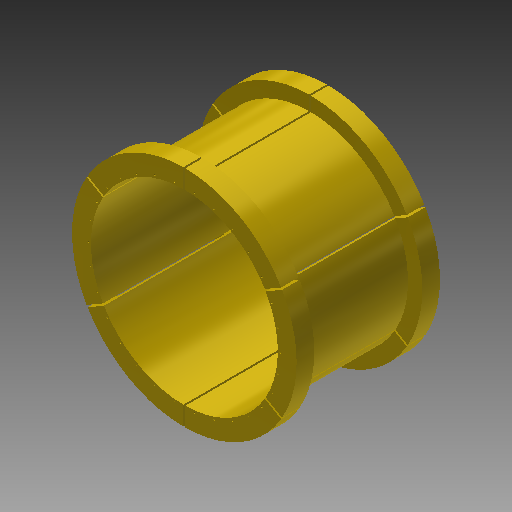
# Autodesk Inventor part: Electrode 4
Saved by Autodesk Inventor 2017 (Build 210142000, 142)
## iProperties
Created: 2009-05-06
Part Number: Electrode 4
Document SubType Name: Modeling
Designer: Serena
Material: Default
Density: 1 g/cm^3
Appearance: Glossy - Gold
Author: Serena
Autodesk Inventor part; units mm, degrees
ref_plane "YZ Plane" through (0, 0, 0) normal (1, 0, 0) x (0, 1, 0)
ref_plane "XZ Plane" through (0, 0, 0) normal (0, 1, 0) x (-1, 0, 0)
ref_plane "XY Plane" through (0, 0, 0) normal (0, 0, 1) x (1, 0, 0)
sketch "Sketch1" plane through (0, 0, 0) normal (0, 0, 1) x (1, 0, 0)
  circle A0 centre (0, 0) radius 100.35
  circle A1 centre (0, 0) radius 105.35
  dimension "d0" = 200.7
  dimension "d1" = 210.7
  constraints: 2 centre point, 1 coincident
  measures "d0" diameter of A0
  measures "d1" diameter of A1
extrude "Extrusion1" add sketch "Sketch1" along normal blind 154
sketch "Sketch2" plane through (0, 0, 154) normal (0, 0, 1) x (1, 0, 0)
  circle A0 centre (0, 0) radius 100.35
  circle A1 centre (0, 0) radius 105.35
  line L0 (0, 0) -> (0, -108.273006)
  line L1 (-1, -100.345017) -> (-1, -105.345254)
  line L2 (1, -100.345017) -> (1, -105.345254)
  line L3 (0, -101.649951) -> (1, -101.649951)
  line L4 (0, -102.197731) -> (-1, -102.197731)
  line L5 (-87.401334, -49.306483) -> (-91.731666, -51.806602)
  line L6 (-86.401334, -51.038534) -> (-90.731666, -53.538652)
  line L7 (-86.401334, 51.038534) -> (-90.731666, 53.538652)
  line L8 (-87.401334, 49.306483) -> (-91.731666, 51.806602)
  line L9 (1, 100.345017) -> (1, 105.345254)
  line L10 (-1, 100.345017) -> (-1, 105.345254)
  line L11 (87.401334, 49.306483) -> (91.731666, 51.806602)
  line L12 (86.401334, 51.038534) -> (90.731666, 53.538652)
  line L13 (86.401334, -51.038534) -> (90.731666, -53.538652)
  line L14 (87.401334, -49.306483) -> (91.731666, -51.806602)
  line L15 (87.401334, 49.306483) -> (91.731666, 51.806602)
  line L16 (86.401334, 51.038534) -> (90.731666, 53.538652)
  line L17 (86.401334, -51.038534) -> (90.731666, -53.538652)
  line L18 (87.401334, -49.306483) -> (91.731666, -51.806602)
  line L19 (-1, -100.345017) -> (-1, -105.345254)
  line L20 (1, -100.345017) -> (1, -105.345254)
  line L21 (-87.401334, -49.306483) -> (-91.731666, -51.806602)
  line L22 (-86.401334, -51.038534) -> (-90.731666, -53.538652)
  line L23 (-86.401334, 51.038534) -> (-90.731666, 53.538652)
  line L24 (-87.401334, 49.306483) -> (-91.731666, 51.806602)
  point P0 (-87.53144, -51.691001)
  point P1 (-89.005831, -50.23284)
  point P2 (-88.53144, 49.95895)
  point P3 (-88.005831, 51.964891)
  point P4 (-1, 101.649951)
  point P5 (1, 102.197731)
  point P6 (87.53144, 51.691001)
  point P7 (89.005831, 50.23284)
  point P8 (88.53144, -49.95895)
  point P9 (88.005831, -51.964891)
  point P10 (89.005831, 50.23284)
  point P11 (87.53144, 51.691001)
  point P12 (88.005831, -51.964891)
  point P13 (88.53144, -49.95895)
  point P14 (-1, -102.197731)
  point P15 (1, -101.649951)
  point P16 (-89.005831, -50.23284)
  point P17 (-87.53144, -51.691001)
  point P18 (-88.005831, 51.964891)
  point P19 (-88.53144, 49.95895)
  dimension "d5" = 1
  dimension "d8" = 360
  dimension "d12" = 360
  constraints: 50 end point, 24 point on line, 4 point on circle, 3 parallel, 2 perpendicular, 1 vertical, 104 other
  measures "d5" distance between parallel lines of L1 L0
sketch "Sketch3" plane through (0, 0, 154) normal (0, 0, 1) x (1, 0, 0)
  circle A0 centre (0, 0) radius 100.35
  circle A1 centre (0, 0) radius 105.35
  line L0 (86.401334, -51.038534) -> (90.731666, -53.538652)
  line L1 (87.401334, -49.306483) -> (91.731666, -51.806602)
  line L2 (86.401334, -51.038534) -> (90.731666, -53.538652)
  line L3 (87.401334, -49.306483) -> (91.731666, -51.806602)
  arc A2 (90.731666, -53.538652) -> (91.731666, -51.806602) centre (1.73213, -1.000046) ccw
  arc A3 (86.401334, -51.038534) -> (87.401334, -49.306483) centre (0, 0) ccw
  constraints: 4 end point, 4 point on circle, 2 centre point, 2 collinear
extrude "Extrusion2" cut sketch "Sketch3" against normal blind 155 contours A0 L1 A1 L0 picked at (88.734946, -50.333043)
pattern_circular "Circular Pattern1" count 6 over 360 about axis through (0, 0, 0) along (0, 0, 1) of "Extrusion2"
sketch "Sketch7" plane through (0, 0, 0) normal (0, 0, -1) x (-1, 0, 0)
  arc A0 (1, -100.345017) -> (86.401334, -51.038534) centre (0, 0) ccw
  circle A1 centre (0, 0) radius 103.35
  circle A2 centre (0, 0) radius 120.65
  dimension "d37" = 206.7
  dimension "d38" = 241.3
  constraints: 2 centre point, 2 coincident
  measures "d37" diameter of A1
  measures "d38" diameter of A2
extrude "Extrusion4" add sketch "Sketch7" against normal blind 18.9992
sketch "Sketch6" plane through (0, 0, 154) normal (0, 0, 1) x (1, 0, 0)
  arc A0 (-91.731666, 51.806602) -> (-91.731666, -51.806602) centre (0, 0) ccw
  circle A1 centre (0, 0) radius 120.65
  circle A2 centre (0, 0) radius 103.35
  dimension "d33" = 241.3
  dimension "d34" = 206.7
  constraints: 2 centre point, 2 coincident
  measures "d33" diameter of A1
  measures "d34" diameter of A2
extrude "Extrusion3" add sketch "Sketch6" against normal blind 18.9992
sketch "Sketch4" plane through (0, 0, 0) normal (0, 1, 0) x (-1, 0, 0)
  line L0 (105.35, 0) -> (105.35, 154)
  line L1 (100.35, 0) -> (100.35, 154)
  line L2 (87.401334, 154) -> (100.35, 154)
  line L3 (91.731666, 154) -> (105.35, 154)
  line L4 (102.85, 154) -> (102.85, 142)
  line L5 (102.85, 154) -> (102.85, 162)
  circle A0 centre (102.85, 154.5) radius 1
  line L6 (102.85, 154) -> (102.85, 153.5)
  line L7 (102.85, 154) -> (101.983975, 154)
  line L8 (102.85, 154) -> (103.716025, 154)
  arc A1 (102.85, 153.5) -> (103.716025, 154) centre (102.85, 154.5) ccw
  arc A2 (101.983975, 154) -> (102.85, 153.5) centre (102.85, 154.5) ccw
  line L9 (-1, 0) -> (-1, 154) construction
  line L10 (-86.401334, 154) -> (-1, 154) construction
  line L11 (-86.401334, 154) -> (-86.401334, 0) construction
  line L12 (-1, 0) -> (-86.401334, 0) construction
  line L13 (1, 0) -> (-1, 0) construction
  line L14 (-1, 154) -> (1, 154) construction
  line L15 (1, 135.0008) -> (-1, 135.0008) construction
  line L16 (0, 154) -> (0, 135.0008) construction
  dimension "d20" = 0.5
  dimension "d21" = 2
  dimension "d53" = 102.85
  constraints: 12 end point, 7 point on circle, 5 point on line, 4 concentric, 3 centre point, 2 midpoint, 1 collinear, 1 perpendicular
  measures "d20" distance of L4.start L6.end
  measures "d21" diameter of A0
  measures "d53" distance between parallel lines of L4 L16
revolve "Revolution1" cut sketch "Sketch4" angle 360 about axis through (-102.85, 0, 154) along (0, 0, -1) picked at (103.38639, 153.943623) contours L3 A0 L4
pattern_circular "Circular Pattern2" count 30 over 360 about axis through (0, 0, 0) along (0, 0, 1) of "Revolution1"
sketch "Sketch5" plane through (0, 0, 0) normal (0, 1, 0) x (-1, 0, 0)
  line L0 (105.35, 0) -> (105.35, 154)
  line L1 (100.35, 0) -> (100.35, 154)
  line L2 (91.731666, 0) -> (105.35, 0)
  line L3 (102.85, 0) -> (102.85, 14)
  line L4 (102.85, 0) -> (102.85, -13)
  circle A0 centre (102.85, -0.5) radius 1
  line L5 (102.85, 0) -> (102.85, 0.5)
  line L6 (102.85, 0) -> (101.983975, 0)
  line L7 (102.85, 0) -> (103.716025, 0)
  arc A1 (103.716025, 0) -> (102.85, 0.5) centre (102.85, -0.5) ccw
  arc A2 (102.85, 0.5) -> (101.983975, 0) centre (102.85, -0.5) ccw
  line L8 (1, 0) -> (-1, 0)
  line L9 (-1, 18.9992) -> (1, 18.9992)
  line L10 (0, 0) -> (0, 18.9992) construction
  dimension "d27" = 0.5
  dimension "d28" = 2
  dimension "d54" = 102.85
  constraints: 12 end point, 7 point on circle, 5 point on line, 3 centre point, 3 concentric, 2 midpoint, 1 collinear, 1 perpendicular
  measures "d27" distance of L3.start L5.end
  measures "d28" diameter of A0
  measures "d54" distance between parallel lines of L10 L3
revolve "Revolution2" cut sketch "Sketch5" angle 360 about axis through (-102.85, 0, 0) along (0, 0, 1) picked at (103.38639, 0.056377) contours L3 A0 L2
pattern_circular "Circular Pattern3" count 30 over 360 about axis through (0, 0, 0) along (0, 0, 1) of "Revolution2"
sketch "Sketch8" plane through (0, 0, 0) normal (0, 0, -1) x (-1, 0, 0)
  circle A0 centre (0, 0) radius 120.65
  line L0 (-1, -103.345162) -> (-1, -100.345017)
  arc A1 (-86.401334, -51.038534) -> (-1, -100.345017) centre (0, 0) ccw
  line L1 (-86.401334, -51.038534) -> (-88.999536, -52.538606)
  arc A2 (-89.999536, -50.806556) -> (-88.999536, -52.538606) centre (0, 0) ccw
  line L2 (-89.999536, -50.806556) -> (-87.401334, -49.306483)
  arc A3 (-87.401334, 49.306483) -> (-87.401334, -49.306483) centre (0, 0) ccw
  line L3 (-87.401334, 49.306483) -> (-89.999536, 50.806556)
  arc A4 (-88.999536, 52.538606) -> (-89.999536, 50.806556) centre (0, 0) ccw
  line L4 (-88.999536, 52.538606) -> (-86.401334, 51.038534)
  arc A5 (-1, 100.345017) -> (-86.401334, 51.038534) centre (0, 0) ccw
  line L5 (-1, 100.345017) -> (-1, 103.345162)
  arc A6 (1, 103.345162) -> (-1, 103.345162) centre (0, 0) ccw
  line L6 (1, 103.345162) -> (1, 100.345017)
  arc A7 (86.401334, 51.038534) -> (1, 100.345017) centre (0, 0) ccw
  line L7 (86.401334, 51.038534) -> (88.999536, 52.538606)
  arc A8 (89.999536, 50.806556) -> (88.999536, 52.538606) centre (0, 0) ccw
  line L8 (89.999536, 50.806556) -> (87.401334, 49.306483)
  arc A9 (87.401334, -49.306483) -> (87.401334, 49.306483) centre (0, 0) ccw
  line L9 (87.401334, -49.306483) -> (89.999536, -50.806556)
  arc A10 (88.999536, -52.538606) -> (89.999536, -50.806556) centre (0, 0) ccw
  line L10 (88.999536, -52.538606) -> (86.401334, -51.038534)
  arc A11 (1, -100.345017) -> (86.401334, -51.038534) centre (0, 0) ccw
  line L11 (1, -100.345017) -> (1, -103.345162)
  arc A12 (-1, -103.345162) -> (1, -103.345162) centre (0, 0) ccw
  line L12 (87.401334, -49.306483) -> (104.982376, -59.456902)
  line L13 (86.401334, -51.038534) -> (103.982376, -61.188953)
  constraints: 4 end point, 2 point on circle, 1 parallel, 1 point on line
extrude "Extrusion5" cut sketch "Sketch8" against normal blind 155 contours L13 A10 L12 A0
sketch "Sketch9" plane through (0, 0, 0) normal (0, 0, -1) x (-1, 0, 0)
  line L0 (87.401334, -49.306483) -> (104.982376, -59.456902)
  arc A0 (104.982376, -59.456902) -> (103.982376, -61.188953) centre (0, 0) ccw
  line L1 (103.982376, -61.188953) -> (86.401334, -51.038534)
  arc A1 (1, -100.345017) -> (86.401334, -51.038534) centre (0, 0) ccw
  line L2 (1, -100.345017) -> (1, -103.345162)
  arc A2 (-1, -103.345162) -> (1, -103.345162) centre (0, 0) ccw
  line L3 (-1, -103.345162) -> (-1, -100.345017)
  arc A3 (-86.401334, -51.038534) -> (-1, -100.345017) centre (0, 0) ccw
  line L4 (-86.401334, -51.038534) -> (-88.999536, -52.538606)
  arc A4 (-89.999536, -50.806556) -> (-88.999536, -52.538606) centre (0, 0) ccw
  line L5 (-89.999536, -50.806556) -> (-87.401334, -49.306483)
  arc A5 (-87.401334, 49.306483) -> (-87.401334, -49.306483) centre (0, 0) ccw
  line L6 (-87.401334, 49.306483) -> (-89.999536, 50.806556)
  arc A6 (-88.999536, 52.538606) -> (-89.999536, 50.806556) centre (0, 0) ccw
  line L7 (-88.999536, 52.538606) -> (-86.401334, 51.038534)
  arc A7 (-1, 100.345017) -> (-86.401334, 51.038534) centre (0, 0) ccw
  line L8 (-1, 100.345017) -> (-1, 103.345162)
  arc A8 (1, 103.345162) -> (-1, 103.345162) centre (0, 0) ccw
  line L9 (1, 103.345162) -> (1, 100.345017)
  arc A9 (86.401334, 51.038534) -> (1, 100.345017) centre (0, 0) ccw
  line L10 (86.401334, 51.038534) -> (88.999536, 52.538606)
  arc A10 (89.999536, 50.806556) -> (88.999536, 52.538606) centre (0, 0) ccw
  line L11 (89.999536, 50.806556) -> (87.401334, 49.306483)
  arc A11 (87.401334, -49.306483) -> (87.401334, 49.306483) centre (0, 0) ccw
  line L12 (1, -100.345017) -> (1, -120.645856)
  line L13 (-1, -100.345017) -> (-1, -120.645856)
  constraints: 4 end point, 2 point on circle, 1 parallel, 1 point on line
extrude "Extrusion6" cut sketch "Sketch9" against normal blind 155 contours L13 A2 L12 A0
sketch "Sketch10" plane through (0, 0, 0) normal (0, 0, -1) x (-1, 0, 0)
  line L0 (-1, -120.645856) -> (-1, -100.345017)
  arc A0 (-86.401334, -51.038534) -> (-1, -100.345017) centre (0, 0) ccw
  line L1 (-86.401334, -51.038534) -> (-88.999536, -52.538606)
  arc A1 (-89.999536, -50.806556) -> (-88.999536, -52.538606) centre (0, 0) ccw
  line L2 (-89.999536, -50.806556) -> (-87.401334, -49.306483)
  arc A2 (-87.401334, 49.306483) -> (-87.401334, -49.306483) centre (0, 0) ccw
  line L3 (-87.401334, 49.306483) -> (-89.999536, 50.806556)
  arc A3 (-88.999536, 52.538606) -> (-89.999536, 50.806556) centre (0, 0) ccw
  line L4 (-88.999536, 52.538606) -> (-86.401334, 51.038534)
  arc A4 (-1, 100.345017) -> (-86.401334, 51.038534) centre (0, 0) ccw
  line L5 (-1, 100.345017) -> (-1, 103.345162)
  arc A5 (1, 103.345162) -> (-1, 103.345162) centre (0, 0) ccw
  line L6 (1, 103.345162) -> (1, 100.345017)
  arc A6 (86.401334, 51.038534) -> (1, 100.345017) centre (0, 0) ccw
  line L7 (86.401334, 51.038534) -> (88.999536, 52.538606)
  arc A7 (89.999536, 50.806556) -> (88.999536, 52.538606) centre (0, 0) ccw
  line L8 (89.999536, 50.806556) -> (87.401334, 49.306483)
  arc A8 (87.401334, -49.306483) -> (87.401334, 49.306483) centre (0, 0) ccw
  line L9 (87.401334, -49.306483) -> (104.982376, -59.456902)
  arc A9 (104.982376, -59.456902) -> (-1, -120.645856) centre (0, 0) ccw
  line L10 (86.401334, 51.038534) -> (103.982376, 61.188953)
  line L11 (87.401334, 49.306483) -> (104.982376, 59.456902)
  constraints: 4 end point, 2 parallel, 2 point on circle
extrude "Extrusion7" cut sketch "Sketch10" against normal blind 155 contours A9 L11 A7 L10
sketch "Sketch11" plane through (0, 0, 0) normal (0, 0, -1) x (-1, 0, 0)
  line L0 (86.401334, 51.038534) -> (103.982376, 61.188953)
  arc A0 (103.982376, 61.188953) -> (-1, -120.645856) centre (0, 0) ccw
  line L1 (-1, -120.645856) -> (-1, -100.345017)
  arc A1 (-86.401334, -51.038534) -> (-1, -100.345017) centre (0, 0) ccw
  line L2 (-86.401334, -51.038534) -> (-88.999536, -52.538606)
  arc A2 (-89.999536, -50.806556) -> (-88.999536, -52.538606) centre (0, 0) ccw
  line L3 (-89.999536, -50.806556) -> (-87.401334, -49.306483)
  arc A3 (-87.401334, 49.306483) -> (-87.401334, -49.306483) centre (0, 0) ccw
  line L4 (-87.401334, 49.306483) -> (-89.999536, 50.806556)
  arc A4 (-88.999536, 52.538606) -> (-89.999536, 50.806556) centre (0, 0) ccw
  line L5 (-88.999536, 52.538606) -> (-86.401334, 51.038534)
  arc A5 (-1, 100.345017) -> (-86.401334, 51.038534) centre (0, 0) ccw
  line L6 (-1, 100.345017) -> (-1, 103.345162)
  arc A6 (1, 103.345162) -> (-1, 103.345162) centre (0, 0) ccw
  line L7 (1, 103.345162) -> (1, 100.345017)
  arc A7 (86.401334, 51.038534) -> (1, 100.345017) centre (0, 0) ccw
  line L8 (-1, 100.345017) -> (-1, 120.645856)
  line L9 (1, 100.345017) -> (1, 120.645856)
  constraints: 4 end point, 2 parallel, 2 point on circle
extrude "Extrusion8" cut sketch "Sketch11" against normal blind 155 contours L9 A6 L8 A0
sketch "Sketch12" plane through (0, 0, 0) normal (0, 0, -1) x (-1, 0, 0)
  line L0 (-1, 100.345017) -> (-1, 120.645856)
  arc A0 (-1, 120.645856) -> (-1, -120.645856) centre (0, 0) ccw
  line L1 (-1, -120.645856) -> (-1, -100.345017)
  arc A1 (-86.401334, -51.038534) -> (-1, -100.345017) centre (0, 0) ccw
  line L2 (-86.401334, -51.038534) -> (-88.999536, -52.538606)
  arc A2 (-89.999536, -50.806556) -> (-88.999536, -52.538606) centre (0, 0) ccw
  line L3 (-89.999536, -50.806556) -> (-87.401334, -49.306483)
  arc A3 (-87.401334, 49.306483) -> (-87.401334, -49.306483) centre (0, 0) ccw
  line L4 (-87.401334, 49.306483) -> (-89.999536, 50.806556)
  arc A4 (-88.999536, 52.538606) -> (-89.999536, 50.806556) centre (0, 0) ccw
  line L5 (-88.999536, 52.538606) -> (-86.401334, 51.038534)
  arc A5 (-1, 100.345017) -> (-86.401334, 51.038534) centre (0, 0) ccw
  line L6 (-87.401334, 49.306483) -> (-104.982376, 59.456902)
  line L7 (-86.401334, 51.038534) -> (-103.982376, 61.188953)
  constraints: 4 end point, 2 parallel, 2 point on circle
extrude "Extrusion9" cut sketch "Sketch12" against normal blind 155 contours L7 A4 L6 A0
sketch "Sketch13" plane through (0, 0, 0) normal (0, 0, -1) x (-1, 0, 0)
  line L0 (-87.401334, 49.306483) -> (-104.982376, 59.456902)
  arc A0 (-104.982376, 59.456902) -> (-1, -120.645856) centre (0, 0) ccw
  line L1 (-1, -120.645856) -> (-1, -100.345017)
  arc A1 (-86.401334, -51.038534) -> (-1, -100.345017) centre (0, 0) ccw
  line L2 (-86.401334, -51.038534) -> (-88.999536, -52.538606)
  arc A2 (-89.999536, -50.806556) -> (-88.999536, -52.538606) centre (0, 0) ccw
  line L3 (-89.999536, -50.806556) -> (-87.401334, -49.306483)
  arc A3 (-87.401334, 49.306483) -> (-87.401334, -49.306483) centre (0, 0) ccw
  line L4 (-86.401334, -51.038534) -> (-103.982376, -61.188953)
  line L5 (-87.401334, -49.306483) -> (-104.982376, -59.456902)
  constraints: 4 end point, 2 parallel, 2 point on circle
extrude "Extrusion10" cut sketch "Sketch13" against normal blind 155 contours L5 A2 L4 A0
equation "\"d38\" = d33"
body "Solid1"
